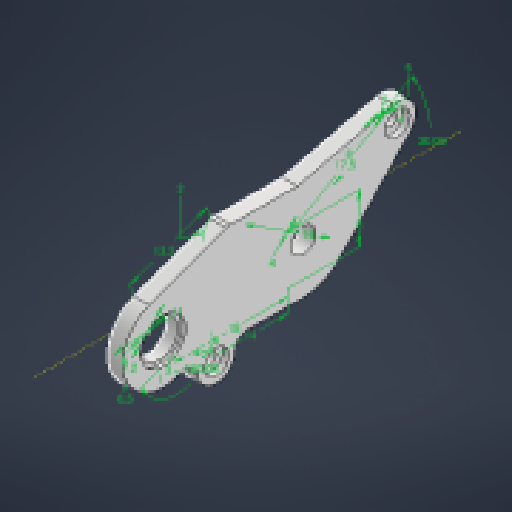
# Autodesk Inventor part: GearCover
Saved by Autodesk Inventor 2024.2 (Build 282272000, 272)
## iProperties
Created: 2023-12-29
Part Number: GearCover
Material: 一般
Document SubType Name: モデリング
Designer: Hanaoka
Density: 1 g/cm^3
Appearance: 既定
Sheet Metal Rule: Default
Author: Hanaoka
Autodesk Inventor part; units mm, degrees
ref_plane "YZ Plane" through (0, 0, 0) normal (1, 0, 0) x (0, 1, 0)
ref_plane "XZ Plane" through (0, 0, 0) normal (0, 1, 0) x (-1, 0, 0)
ref_plane "XY Plane" through (0, 0, 0) normal (0, 0, 1) x (1, 0, 0)
sketch "スケッチ1" plane through (0, 0, 0) normal (1, 0, 0) x (0, 1, 0)
  circle A0 centre (-2.7433, 22.562) radius 3.6
  circle A1 centre (-2.7433, 22.562) radius 3
  arc A2 (3.3647, 24.7851) -> (-8.8513, 20.3389) centre (-2.7433, 22.562) ccw
  line L0 (-8.8513, 20.3389) -> (-8.1809, 18.4971)
  line L1 (-8, 17.471) -> (-8, 0)
  line L2 (8, 0) -> (8, 11.6972)
  line L3 (7.8794, 12.3812) -> (3.3647, 24.7851)
  arc A3 (8, 11.6972) -> (7.8794, 12.3812) centre (6, 11.6972) ccw
  arc A4 (-8, 0) -> (8, 0) centre (0, 0) ccw
  circle A5 centre (0, 0) radius 2
  line L4 (-8, 18) -> (-8, 0) construction
  line L5 (-8, 0) -> (0, 0) construction
  line L6 (0, -27.9652) -> (0, 40.7029) construction
  arc A6 (-8, 17.471) -> (-8.1809, 18.4971) centre (-11, 17.471) ccw
  circle A7 centre (8.75, -15.1554) radius 3
  line L7 (0, 0) -> (8.75, -15.1554) construction
  circle A8 centre (0, 0) radius 8 construction
  line L8 (-5.4965, -5.8127) -> (6.6888, -17.3352)
  line L9 (11.6683, -14.4603) -> (7.7823, 1.8538)
  circle A9 centre (8.75, -15.1554) radius 2
  circle A10 centre (8.75, -15.1554) radius 1
  circle A11 centre (-2.7433, 22.562) radius 5.5 construction
  line L10 (2.7536, 22.3772) -> (1.9989, -0.0672) construction
  line L11 (-8.0357, 21.0653) -> (-1.9245, -0.5443) construction
  circle A12 centre (-10, 14) radius 2
  circle A13 centre (-10, 14) radius 1
  circle A14 centre (-10, 14) radius 3
  point P0 (8, 12.0498)
  point P1 (8, 0.9397)
  point P2 (-5.4965, -5.8127)
  point P3 (-8, 16.2361)
  point P4 (-8, 11.7639)
  point P5 (-8, 14)
  dimension "d0" = 6
  dimension "d1" = 7.2
  dimension "d2" = 6.5
  dimension "d9" = 2
  dimension "d13" = 160
  dimension "d14" = 8
  dimension "d15" = 4
  dimension "d18" = 13.2
  dimension "d19" = 8
  dimension "d20" = 18
  dimension "d26" = 3
  dimension "d55" = 6
  dimension "d56" = 17.5
  dimension "d58" = 30
  dimension "d59" = 16
  dimension "d60" = 4
  dimension "d61" = 2
  dimension "d75" = 11
  dimension "d78" = 6
  dimension "d79" = 4
  dimension "d80" = 2
  dimension "d81" = 14
  constraints: 22 end point, 17 tangent, 16 point on circle, 15 centre point, 11 coincident, 4 point on line, 2 parallel, 1 perpendicular, 1 vertical
  measures "d0" diameter of A1
  measures "d1" diameter of A0
  measures "d2" radius of A2
  measures "d9" radius of A3
  measures "d13" angle of L1 L0
  measures "d14" radius of A4
  measures "d15" diameter of A5
  measures "d18" distance of L3.start L3.end
  measures "d19" distance of L4.end L5.end
  measures "d20" distance of L4.start L4.end
  measures "d26" radius of A6
  measures "d55" diameter of A7
  measures "d56" distance of L7.start L7.end
  measures "d58" angle of L6 L7
  measures "d59" diameter of A8
  measures "d60" diameter of A9
  measures "d61" diameter of A10
  measures "d75" diameter of A11
  measures "d78" diameter of A14
  measures "d79" diameter of A12
  measures "d80" diameter of A13
  measures "d81" vertical distance of L1.end A12.centre
extrude "押し出し3" add sketch "スケッチ1" along normal blind 2.5 contours A0 | L3 A3 L2 A4 L1 A14 A6 L0 A2 | L9 A7 L8 A4 L2 | A14 L1 | L1 A14 | A7
sketch "スケッチ2" plane through (2.5, 0, 0) normal (1, 0, 0) x (0, 0, -1)
  line L0 (-0.9397, 8) -> (-11.6972, 8) projected
  arc A0 (-11.6972, 8) -> (-12.3812, 7.8794) centre (-11.6972, 6) ccw projected
  line L1 (-12.3812, 7.8794) -> (-24.7851, 3.3647) projected
  arc A1 (-24.7851, 3.3647) -> (-20.3389, -8.8513) centre (-22.562, -2.7433) ccw projected
  line L2 (-20.3389, -8.8513) -> (-18.4971, -8.1809) projected
  arc A2 (-17.471, -8) -> (-18.4971, -8.1809) centre (-17.471, -11) ccw projected
  line L3 (-17.471, -8) -> (-16.2361, -8) projected
  arc A3 (0, -8) -> (5.8127, -5.4965) centre (0, 0) ccw projected
  circle A4 centre (-22.562, -2.7433) radius 3 projected
  circle A5 centre (-22.562, -2.7433) radius 3.6
  line L4 (5.8127, -5.4965) -> (17.3352, 6.6888) projected
  arc A6 (17.3352, 6.6888) -> (14.4603, 11.6683) centre (15.1554, 8.75) ccw projected
  line L5 (14.4603, 11.6683) -> (-0.9397, 8) projected
  arc A7 (-16.2361, -8) -> (-11.7639, -8) centre (-14, -10) ccw projected
  line L6 (-11.7639, -8) -> (0, -8) projected
  dimension "d32" = 7.2
  constraints: 1 centre point, 1 coincident
  measures "d32" diameter of A5
extrude "押し出し4" cut sketch "スケッチ2" against normal blind 0.6 contours A5
extrude "押し出し5" add sketch "スケッチ1" along normal blind 1.5 contours A12 | A9
fillet "フィレット1" radius 2 2 edges at (1.25, -8, 11.7639) (1.25, -8, 16.2361)
